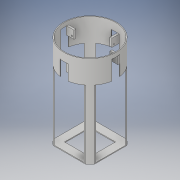
# Autodesk Inventor part: Hull
Saved by Autodesk Inventor 2018 (Build 220112000, 112)
## iProperties
Created: 2017-12-27
Part Number: Hull
Material: Generic
Document SubType Name: Modeling
Designer: Suchanek
Density: 1 g/cm^3
Appearance: Default
Mass: 15.1041 g
Surface Area: 312.787 cm^2
Volume: 15.1041 cm^3
Author: Suchanek
Autodesk Inventor part; units mm, degrees
ref_plane "YZ Plane" through (0, 0, 0) normal (1, 0, 0) x (0, 1, 0)
ref_plane "XZ Plane" through (0, 0, 0) normal (0, 1, 0) x (-1, 0, 0)
ref_plane "XY Plane" through (0, 0, 0) normal (0, 0, 1) x (1, 0, 0)
sketch "Sketch1" plane through (0, 0, 0) normal (0, 0, 1) x (1, 0, 0)
  line L0 (0, 0) -> (33, 0)
  line L1 (33, 0) -> (33, 1)
  line L2 (33, 1) -> (0, 1)
  line L3 (0, 1) -> (0, 0)
  line L4 (33, 0) -> (32, 0)
  line L5 (32, 0) -> (32, 115)
  line L6 (32, 115) -> (33, 115)
  line L7 (33, 115) -> (33, 0)
  line L8 (33, 115) -> (0, 115)
  line L9 (0, 115) -> (0, 115)
  line L10 (0, 115) -> (33, 115)
  line L11 (33, 115) -> (33, 115)
  line L12 (0, 115) -> (0, 1)
  line L13 (-5, 105) -> (5, 105)
  line L14 (5, 105) -> (5, 5)
  line L15 (5, 5) -> (-5, 5)
  line L16 (-5, 5) -> (-5, 105)
  dimension "d0" = 33
  dimension "d1" = 1
  dimension "d2" = 1
  dimension "d3" = 115
  dimension "d4" = 33
  dimension "d5" = 0
  dimension "d6" = 10
  dimension "d7" = 100
  dimension "d8" = 4
  constraints: 34 end point, 8 equal length, 4 perpendicular, 3 horizontal, 1 other
  measures "d0" distance of L2.end L1.end
  measures "d1" distance of L1.end L0.end
  measures "d2" distance of L5.end L6.end
  measures "d3" distance of L4.end L5.end
  measures "d4" distance of L10.end L9.end
  measures "d5" distance of L9.end L8.end
  measures "d6" distance of L14.end L15.end
  measures "d7" distance of L15.end L13.start
  measures "d8" distance from line of L1.end L15
sketch "Sketch2" plane through (0, 0, 0) normal (1, 0, 0) x (0, 1, 0)
  line L0 (105, 5) -> (5, 5)
  line L1 (5, 5) -> (5, -5)
  line L2 (5, -5) -> (105, -5)
  line L3 (105, -5) -> (105, 5)
  line L4 (0, 0) -> (0, -10)
  line L5 (0, 0) -> (115, 0)
  dimension "d9" = 10
  dimension "d10" = 5
  dimension "d12" = 115
  dimension "d13" = 10
  dimension "d14" = 100
  constraints: 12 end point, 2 horizontal, 2 parallel, 1 perpendicular, 1 vertical, 1 other
  measures "d9" distance of L4.start L4.end
  measures "d10" distance between parallel lines of L1 L4
  measures "d12" distance of L4.start L5.end
  measures "d13" distance between parallel lines of L0 L2
  measures "d14" distance of L1.end L2.end
extrude "Extrusion1" add sketch "Sketch2" along normal mid plane 10
revolve "Revolution1" add sketch "Sketch1" angle 360 about axis through (0, 115, 0) along (0, -1, 0) contours L3 L2 L5 L0 | L5 L2 L1 L0 | L5 L6 L7 L2
sketch "Sketch3" plane through (-5, 5, 5) normal (0, 0, 1) x (1, 0, 0)
  line L0 (0, 100) -> (10, 100) projected
  line L1 (10, 100) -> (10, 0) projected
  line L2 (0, 100) -> (10, 100)
  line L3 (10, 100) -> (10, 0)
  line L4 (10, 0) -> (0, 0)
  line L5 (0, 0) -> (0, 100)
  point P0 (5, -5)
  dimension "d18" = 100
  constraints: 8 end point, 2 parallel, 1 horizontal, 1 perpendicular
  measures "d18" distance of L2.end L1.end
extrude "Extrusion2" cut sketch "Sketch3" along normal mid plane 200
sketch "Sketch4" plane through (5, 0, 0) normal (1, 0, 0) x (0, 0, -1)
  line L0 (-5, 110) -> (-5, 5) projected
  line L1 (-5, 110) -> (5, 110)
  line L2 (5, 110) -> (5, 5)
  line L3 (5, 5) -> (-5, 5)
  line L4 (-5, 5) -> (-5, 110)
  point P0 (0, 0)
  dimension "d21" = 10
  constraints: 8 end point, 2 parallel, 1 horizontal, 1 perpendicular, 1 point on line
  measures "d21" distance of L2.end L3.end
extrude "Extrusion3" cut sketch "Sketch4" along normal mid plane 200
sketch "Sketch5" plane through (-32.619, 5, -5) normal (0, 0, 1) x (1, 0, 0)
  line L0 (65.238, 105) -> (64.226, 105) projected
  line L1 (65.238, 105) -> (55.238, 105)
  line L2 (55.238, 105) -> (55.238, 95)
  line L3 (55.238, 95) -> (65.238, 95)
  line L4 (65.238, 95) -> (65.238, 105)
  line L5 (0, 105) -> (-0.381, 105) projected
  line L6 (0, 105) -> (10, 105)
  line L7 (10, 105) -> (10, 95)
  line L8 (10, 95) -> (0, 95)
  line L9 (0, 95) -> (0, 105)
  circle A0 centre (7.5, 97.5) radius 1
  circle A1 centre (57.738, 97.5) radius 1
  point P0 (32.619, -5)
  dimension "d26" = 10
  dimension "d27" = 10
  dimension "d56" = 10
  dimension "d57" = 10
  dimension "d58" = 2
  dimension "d59" = 2.5
  dimension "d60" = 2.5
  dimension "d61" = 2
  dimension "d62" = 2.5
  dimension "d63" = 2.5
  constraints: 16 end point, 4 parallel, 2 centre point, 2 horizontal, 2 perpendicular
  measures "d26" distance of L3.end L2.end
  measures "d27" distance of L2.end L1.end
  measures "d56" distance of L7.end L8.end
  measures "d57" distance of L6.end L7.end
  measures "d58" diameter of A0
  measures "d59" distance from line of L7 A0.centre
  measures "d60" distance from line of L8 A0.centre
  measures "d61" diameter of A1
  measures "d62" distance from line of A1.centre L2
  measures "d63" distance from line of A1.centre L3
extrude "Extrusion4" add sketch "Sketch5" along normal blind 2.5
sketch "Sketch6" plane through (5, 5, 31.607) normal (-1, 0, 0) x (0, 0, 1)
  line L0 (0, 100) -> (1.0121, 100) projected
  line L1 (1.0121, 100) -> (-8.9879, 100)
  line L2 (-8.9879, 100) -> (-8.9879, 90)
  line L3 (-8.9879, 90) -> (1.0121, 90)
  line L4 (1.0121, 90) -> (1.0121, 100)
  line L5 (-64.226, 100) -> (-63.2139, 100) projected
  line L6 (-64.226, 100) -> (-54.226, 100)
  line L7 (-54.226, 100) -> (-54.226, 90)
  line L8 (-54.226, 90) -> (-64.226, 90)
  line L9 (-64.226, 90) -> (-64.226, 100)
  circle A0 centre (-6.4879, 92.5) radius 1
  circle A1 centre (-56.726, 92.5) radius 1
  point P0 (-31.607, -5)
  dimension "d30" = 10
  dimension "d31" = 10
  dimension "d32" = 10
  dimension "d33" = 10
  dimension "d64" = 2
  dimension "d65" = 2.5
  dimension "d66" = 2.5
  dimension "d67" = 2
  dimension "d68" = 2.5
  dimension "d69" = 1.5
  constraints: 16 end point, 4 parallel, 2 centre point, 2 horizontal, 2 perpendicular
  measures "d30" distance of L3.end L2.end
  measures "d31" distance of L2.end L1.end
  measures "d32" distance of L7.end L8.end
  measures "d33" distance of L6.end L7.end
  measures "d64" diameter of A0
  measures "d65" distance from line of L2 A0.centre
  measures "d66" distance from line of L3 A0.centre
  measures "d67" diameter of A1
  measures "d68" distance from line of L7 A1.centre
  measures "d69" distance edge to line of A1 L8
extrude "Extrusion5" add sketch "Sketch6" along normal blind 2.5
sketch "Sketch7" plane through (0, 1, 0) normal (0, 1, 0) x (1, 0, 0)
  line L0 (0, 0) -> (-26, 0)
  line L1 (-26, 0) -> (-26, 26)
  line L2 (-26, 26) -> (0, 26)
  line L3 (0, 26) -> (0, 0)
  line L4 (-26, 26) -> (26, 26)
  line L5 (26, 26) -> (26, 33)
  line L6 (26, 33) -> (-26, 33)
  line L7 (-26, 33) -> (-26, 26)
  line L8 (26, 26) -> (33, 26)
  line L9 (33, 26) -> (33, -26)
  line L10 (33, -26) -> (26, -26)
  line L11 (26, -26) -> (26, 26)
  line L12 (-26, 26) -> (-33, 26)
  line L13 (-33, 26) -> (-33, -26)
  line L14 (-33, -26) -> (-26, -26)
  line L15 (-26, -26) -> (-26, 26)
  line L16 (-26, -26) -> (26, -26)
  line L17 (26, -26) -> (26, -33)
  line L18 (26, -33) -> (-26, -33)
  line L19 (-26, -33) -> (-26, -26)
  dimension "d36" = 26
  dimension "d37" = 26
  dimension "d38" = 52
  dimension "d39" = 7
  dimension "d40" = 7
  dimension "d41" = 52
  dimension "d42" = 7
  dimension "d43" = 52
  dimension "d44" = 52
  dimension "d45" = 7
  constraints: 40 end point, 10 parallel, 5 horizontal, 5 perpendicular
  measures "d36" distance of L1.end L2.end
  measures "d37" distance of L0.end L1.end
  measures "d38" distance of L6.end L5.end
  measures "d39" distance of L5.end L4.end
  measures "d40" distance of L9.end L10.end
  measures "d41" distance of L8.end L9.end
  measures "d42" distance of L14.end L13.end
  measures "d43" distance of L13.end L12.end
  measures "d44" distance of L17.end L18.end
  measures "d45" distance of L16.end L17.end
extrude "Extrusion6" cut sketch "Sketch7" along normal blind 85 and the other way blind 5 contours L15 L14 L13 L12 L1 | L2 L7 L6 L5 L4 | L16 L17 L18 L19 | L8 L9 L10 L11
sketch "Sketch8" plane through (-18.6548, 1, 26) normal (0, 1, 0) x (1, 0, 0)
  point P0 (18.6548, 26)
sketch "Sketch9" plane through (-18.6548, 1, 26) normal (0, 1, 0) x (1, 0, 0)
  line L0 (2.6548, 42) -> (34.6548, 42)
  line L1 (34.6548, 42) -> (34.6548, 10)
  line L2 (34.6548, 10) -> (2.6548, 10)
  line L3 (2.6548, 10) -> (2.6548, 42)
  line L4 (37.3095, 52) -> (0, 52) projected
  line L5 (-7.3452, 5.6776) -> (-7.3452, 46.3224) projected
  line L6 (0, 0) -> (37.3095, 0) projected
  line L7 (44.6548, 7.3452) -> (44.6548, 44.6548) projected
  point P0 (18.6548, 26)
  dimension "d50" = 10
  dimension "d51" = 10
  dimension "d52" = 10
  dimension "d53" = 10
  constraints: 8 end point, 2 parallel, 1 horizontal, 1 perpendicular
  measures "d50" distance between parallel lines of L4 L0
  measures "d51" distance between parallel lines of L5 L3
  measures "d52" distance between parallel lines of L6 L2
  measures "d53" distance between parallel lines of L7 L1
extrude "Extrusion7" cut sketch "Sketch9" against normal blind 10
body "Solid1"
